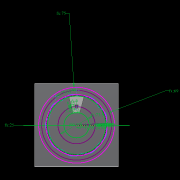
# Autodesk Inventor part: Section_Left_OuterBearing_TBS
Saved by Autodesk Inventor 2022.2 (Build 262287010, 287A)
## iProperties
Created: 2022-05-21
Part Number: Section_Left_OuterBearing_TBS
Material: Generic
Document SubType Name: Modeling
Designer: Árni Þór Þorgeirsson
Density: 1 g/cm^3
Appearance: Default
Author: Árni Þór Þorgeirsson
Autodesk Inventor part; units mm, degrees
ref_plane "YZ Plane" through (0, 0, 0) normal (1, 0, 0) x (0, 1, 0)
ref_plane "XZ Plane" through (0, 0, 0) normal (0, 1, 0) x (-1, 0, 0)
sketch "Sketch1" plane through (0, 0, 0) normal (0, 0, 1) x (1, 0, 0)
  circle A0 centre (0, 0) radius 59.2469 construction
  line L0 (0, 0) -> (59.2469, 0)
  line L1 (0, 0) -> (59.2469, 4.025)
  line L2 (59.2469, 0) -> (59.2469, 4.025)
  circle A1 centre (0, 0) radius 75
  point P0 (56.8, 0)
  dimension "d56" = 59.2469
  dimension "d57" = 4.025
  dimension "d400" = 75
  dimension "d495" = 2.5
  dimension "d496" = 8
  dimension "d531" = 5.5
  dimension "d532" = 5.5
  dimension "d533" = 5.5
  dimension "d537" = 24.5
  dimension "d538" = 3
  dimension "d543" = 5.5
  dimension "d549" = 3
  dimension "d550" = 3
  dimension "d567" = 5.5
  dimension "d568" = 5.5
  constraints: 1 other
sketch "Sketch7" plane through (0, 0, 0) normal (0, 1, 0) x (-1, 0, 0)
  line L0 (0, 0) -> (0, 61.9844)
  line L1 (0, 0) -> (-59.2469, 0) construction
  line L2 (0, 61.9844) -> (-59.2469, 0) construction
  line L3 (0, 61.9844) -> (-64.8494, 0) construction
  line L4 (0, 61.9844) -> (-58.9939, -5.5968) construction
  line L5 (0, 0) -> (0, -61.9844)
  line L6 (0, -61.9844) -> (-59.2469, 0) construction
  line L7 (0, -61.9844) -> (-64.8494, 0) construction
  line L8 (0, -61.9844) -> (-58.9939, 5.5968) construction
  line L9 (-58.9939, 5.5968) -> (-64.8494, 0) construction
  line L10 (-54.1083, 0) -> (-62.8579, -8.363) construction
  line L11 (-54.1083, 0) -> (-38.773, -14.6579) construction
  line L12 (0, -94.3812) -> (0, 132.3969) projected
  line L13 (-75, -5.9919) -> (-75, 6.008)
  line L14 (105, 0) -> (-105, 0) projected
  line L15 (-62.0481, 2.6775) -> (-56.4456, -2.6775) construction
  line L16 (-56.4456, 2.6775) -> (-62.0481, -2.6775) construction
  line L17 (-26.151, -15.9303) -> (-40.3783, -15.9303) construction
  line L18 (-40.3783, -15.9303) -> (-40.3783, -12.7539) construction
  line L19 (-40.3783, -12.7539) -> (-26.151, -12.7539) construction
  line L20 (-26.151, -12.7539) -> (-26.151, -15.9303) construction
  point P0 (-75, 0)
  dimension "Roller_Side_difference" = -0.0002
  dimension "d90" = 61.9844
  dimension "d201" = 75
  dimension "d343" = 92.587
  dimension "d344" = 92.588
  dimension "d367" = 8.1
  constraints: 28 end point, 9 point on line, 3 midpoint, 3 vertical, 2 horizontal, 2 parallel, 2 perpendicular, 1 collinear, 1 symmetric about line, 2 other
  measures "d90" distance of L0.start L0.end
  measures "d201" distance between parallel lines of L5 L13
  measures "d343" angle of L10 L8
  measures "d344" angle of L7 L10
  measures "d367" distance of L3.end L8.end
sketch "Roller1" plane through (0, 0, 0) normal (0, 1, 0) x (-1, 0, 0)
  line L0 (0, 61.9844) -> (-58.9939, -5.5968) construction
  line L1 (0, 61.9844) -> (-64.8494, 0) construction
  line L2 (-54.1083, 0) -> (-38.773, -14.6579) construction
  line L3 (0, -61.9844) -> (-64.8494, 0) construction
  line L4 (-54.0606, 0.0927) -> (-58.9462, -5.5041)
  line L5 (-58.9462, -5.5041) -> (-64.7589, 0.0519)
  line L6 (-64.7589, 0.0519) -> (-59.3884, 5.1851)
  line L7 (-59.3884, 5.1851) -> (-54.0606, 0.0927)
  line L8 (-56.0019, 1.9482) -> (-61.1299, -3.4168)
  line L9 (-61.8526, -2.7261) -> (-56.7246, 2.639)
  point P0 (0, 0)
  dimension "d345" = 0.025
  dimension "d346" = 0.025
  dimension "d347" = 0.1
  dimension "d348" = 0.1
  dimension "d349" = 272.588
  dimension "d350" = 272.587
  dimension "d617" = 0.9997
  constraints: 12 end point, 4 parallel, 3 point on line, 1 midpoint, 1 perpendicular
  measures "d345" distance between parallel lines of L0 L4
  measures "d346" distance between parallel lines of L1 L6
  measures "d347" distance between parallel lines of L3 L5
  measures "d348" distance between parallel lines of L2 L7
  measures "d617" distance between parallel lines of L9 L8
sketch "Roller2" plane through (0, 0, 0) normal (0, 1, 0) x (-1, 0, 0)
  line L0 (0, -61.9844) -> (-58.9939, 5.5968) construction
  line L1 (-54.1083, 0) -> (-62.8579, -8.363) construction
  line L2 (0, -61.9844) -> (-64.8494, 0) construction
  line L3 (0, 61.9844) -> (-64.8494, 0) construction
  line L4 (-58.9956, 5.5606) -> (-54.1429, 0.0016)
  line L5 (-54.1429, 0.0016) -> (-59.4789, -5.0987)
  line L6 (-59.4789, -5.0987) -> (-64.8132, 0)
  line L7 (-64.8132, 0) -> (-58.9956, 5.5606)
  line L8 (-61.9044, 2.7803) -> (-56.8109, -2.5486)
  line L9 (-61.1815, 3.4713) -> (-56.088, -1.8576)
  point P0 (0, 0)
  dimension "d351" = 0.025
  dimension "d352" = 0.025
  dimension "d354" = 0.025
  dimension "d355" = 92.587
  dimension "d356" = 92.588
  dimension "d370" = 0.025
  dimension "d371" = 1
  constraints: 12 end point, 5 parallel, 3 point on line, 1 midpoint, 1 perpendicular
  measures "d351" distance between parallel lines of L0 L4
  measures "d352" distance between parallel lines of L2 L6
  measures "d354" distance between parallel lines of L1 L5
  measures "d355" angle of L5 L4
  measures "d356" angle of L6 L5
  measures "d370" distance from line of L3 L8.start
  measures "d371" distance between parallel lines of L9 L8
sketch "Sketch22" plane through (0, 0, 0) normal (0, 1, 0) x (-1, 0, 0)
  line L0 (-31.756, 8.0215) -> (-17.5287, 8.0215) construction
  line L1 (-17.5287, 8.0215) -> (-17.5287, 4.8451) construction
  line L2 (-17.5287, 4.8451) -> (-31.756, 4.8451) construction
  line L3 (-31.756, 4.8451) -> (-31.756, 8.0215) construction
  point P0 (0, 0)
  dimension "Roller_Side_difference" = -0.0002
  constraints: 2 other
sketch "Sketch2" plane through (0, 0, 0) normal (0, 1, 0) x (-1, 0, 0)
  line L0 (0, 0) -> (0, 59.2469) construction
  line L1 (0, 0) -> (-59.2469, 0) projected
  line L2 (0, 0) -> (0, -59.2469)
  line L3 (0, -59.2469) -> (-59.2469, 0) construction
  line L4 (0, 59.2469) -> (-59.2469, 0) construction
  line L5 (-50.4879, 53.555) -> (0, 59.2469) construction
  line L6 (-29.7354, 7.189) -> (0, 59.2469) construction
  line L7 (-29.7354, 7.189) -> (0, -59.2469) construction
  line L8 (-48.8381, -26.254) -> (0, -59.2469) construction
  point P0 (-40.4258, 18.8211)
  constraints: 16 end point, 3 point on line, 1 perpendicular, 1 symmetric about line, 1 vertical
sketch "Sketch23" plane through (0, 0, 0) normal (0, 1, 0) x (-1, 0, 0)
  line L0 (0, -61.9844) -> (-58.9939, 5.5968) construction
  line L1 (0, -61.9844) -> (-64.8494, 0) construction
  line L2 (0, 61.9844) -> (-58.9939, -5.5968) construction
  line L3 (-58.9939, 5.5968) -> (-64.8494, 0) construction
  line L4 (0, 61.9844) -> (-64.8494, 0) construction
  line L5 (-58.9939, 5.5968) -> (-58.9939, -5.5968) construction
  line L6 (105, 0) -> (-105, 0) projected
  line L7 (-57.6514, 4.0968) -> (-54.1326, 0.0658)
  line L8 (-54.1326, -0.0658) -> (-57.6514, -4.0968)
  line L9 (-60.5995, 4.0968) -> (-64.81, 0.0723)
  line L10 (-64.81, -0.0723) -> (-60.5995, -4.0968)
  arc A0 (-64.81, 0.0723) -> (-64.81, -0.0723) centre (-64.7409, 0) ccw
  arc A1 (-54.1326, -0.0658) -> (-54.1326, 0.0658) centre (-54.2079, 0) ccw
  line L11 (-57.6514, 4.0968) -> (-57.6514, 5.5968)
  line L12 (-57.6514, 5.5968) -> (-25, 5.5968)
  line L13 (-25, 5.5968) -> (-25, -5.5968)
  line L14 (-25, -5.5968) -> (-57.6514, -5.5968)
  line L15 (-57.6514, -5.5968) -> (-57.6514, -4.0968)
  line L16 (-60.5995, 4.0968) -> (-60.5995, 5.5968)
  line L17 (-60.5995, 5.5968) -> (-75, 5.5968)
  line L18 (-75, 5.5968) -> (-75, -5.5968)
  line L19 (-60.5995, -4.0968) -> (-60.5995, -5.5968)
  line L20 (-60.5995, -5.5968) -> (-75, -5.5968)
  line L21 (-58.9939, 5.5968) -> (-58.9939, 5.5968)
  line L22 (-58.9939, -5.5968) -> (-58.9939, -5.5968)
  line L23 (0, -94.3812) -> (0, 132.3969) projected
  line L24 (-64.8856, 0) -> (-75, 0)
  point P0 (0, 0)
  point P1 (-54.0752, 0)
  point P2 (-64.8409, 0)
  point P3 (-75, 0)
  dimension "d378" = 90
  dimension "d379" = 0.1
  dimension "d380" = 0.025
  dimension "d381" = 0.025
  dimension "d382" = 0.025
  dimension "d383" = 0.025
  dimension "d384" = 11.1935
  dimension "d385" = 0
  dimension "d386" = 0
  dimension "d391" = 25
  dimension "d392" = 75
  dimension "d393" = 1.5
  dimension "d394" = 1.5
  dimension "d395" = 1.5
  dimension "d396" = 1.5
  constraints: 36 end point, 10 point on line, 9 vertical, 4 horizontal, 4 parallel, 4 point on circle, 4 tangent, 2 centre point, 1 equal radius, 1 midpoint
  measures "d378" angle of L6 L5
  measures "d379" radius of A0
  measures "d380" distance between parallel lines of L9 L4
  measures "d381" distance between parallel lines of L10 L1
  measures "d382" distance between parallel lines of L0 L7
  measures "d383" distance between parallel lines of L2 L8
  measures "d384" distance of L0.end L2.end
  measures "d385" distance of L2.end L22.end
  measures "d386" distance of L0.end L21.end
  measures "d391" distance between parallel lines of L23 L13
  measures "d392" distance between parallel lines of L18 L23
  measures "d393" distance of L9.start L16.end
  measures "d394" distance of L7.start L11.end
  measures "d395" distance of L14.end L8.end
  measures "d396" distance of L10.end L19.end
revolve "RevRoller1" [suppressed]
fillet "Fillet1" [suppressed]
sketch "Sketch48" plane through (56.7246, 0, 2.639) normal (-0.691, 0, 0.7229) x (0.7229, 0, 0.691)
  line L0 (-2.5, 0.25) -> (2.5, 0.25)
  line L1 (2.5, 0.25) -> (2.5, -0.25)
  line L2 (2.5, -0.25) -> (-2.5, -0.25)
  line L3 (-2.5, -0.25) -> (-2.5, 0.25)
  line L4 (-2.5, 0.25) -> (2.5, -0.25) construction
  line L5 (2.5, 0.25) -> (-2.5, -0.25) construction
  line L6 (-0.25, -2.5) -> (0.25, -2.5)
  line L7 (0.25, -2.5) -> (0.25, 2.5)
  line L8 (0.25, 2.5) -> (-0.25, 2.5)
  line L9 (-0.25, 2.5) -> (-0.25, -2.5)
  line L10 (-0.25, -2.5) -> (0.25, 2.5) construction
  line L11 (0.25, -2.5) -> (-0.25, 2.5) construction
  point P0 (-42.8293, 0)
  point P1 (0, 0)
  point P2 (-0.25, 0.25)
  point P3 (-0.25, -0.25)
  point P4 (0.25, -0.25)
  point P5 (0.25, 0.25)
  dimension "d621" = 5
  dimension "d622" = 0.5
  dimension "d623" = 0.5
  dimension "d624" = 5
  constraints: 24 end point, 4 midpoint, 4 parallel, 2 horizontal, 2 perpendicular
  measures "d621" distance of L1.end L2.end
  measures "d622" distance of L0.end L1.end
  measures "d623" distance of L8.end L7.end
  measures "d624" distance of L7.end L6.end
extrude "Extrusion39" [suppressed]
sketch "Sketch40" plane through (0, 0, -5.231) normal (0, 0, -1) x (-1, 0, 0)
  circle A0 centre (53.5, 0) radius 2.75 projected
  circle A1 centre (0, 0) radius 53.5 projected
  point P0 (53.4293, 2.7491)
  point P1 (53.4293, -2.7491)
  dimension "d585" = 8
  dimension "d587" = 1.75
  dimension "d589" = 3
  dimension "d592" = 2
  dimension "d593" = 12
  dimension "d594" = 12
  dimension "d611" = 360
  constraints: 18 point on circle, 10 centre point, 8 end point, 2 midpoint, 1 horizontal alignment, 1 vertical, 29 other
  measures "d589" diameter of A1
pattern_circular "Circular Pattern13" [suppressed]
feature "Move Body7" [suppressed]
revolve "Revolution13" [suppressed]
fillet "Fillet3" [suppressed]
pattern_circular "Circular Pattern14" [suppressed]
feature "Move Body6" [suppressed]
revolve "Revolution14" add sketch "Sketch23" angle 360 about axis through (0, 0, -10) along (0, 0, 1) contours A1 L7 L11 L12 L13 L6 | L6 L13 L14 L15 L8 A1
revolve "OuterRim_Top2" [suppressed]
revolve "OuterRim_Bottom2" [suppressed]
ref_plane "Work Plane8" through (0, 0, 20) normal (0, 0, 1) x (1, 0, 0)
sketch "Sketch49" plane through (0, 0, 20) normal (0, 0, 1) x (1, 0, 0)
  circle A0 centre (0, 0) radius 75 projected
  circle A1 centre (0, 0) radius 60.5995 projected
  circle A2 centre (0, 0) radius 57.6514 projected
  circle A3 centre (0, 0) radius 25 projected
  circle A4 centre (0, 0) radius 69
  circle A5 centre (0, 0) radius 36.75
  point P0 (0, 69)
  point P1 (0, 36.75)
  point P2 (-40.5572, 55.8222)
  dimension "d629" = 69
  dimension "d630" = 73.5
  dimension "d649" = 36
  constraints: 2 coincident, 2 vertical alignment, 6 other
sketch "Sketch50" plane through (0, 0, 5.5968) normal (0, 0, 1) x (1, 0, 0)
  point P0 (0, 0)
  point P1 (0, 69)
sketch "Sketch51" plane through (0, 0, -5.5968) normal (0, 0, -1) x (-1, 0, 0)
  circle A0 centre (0, 0) radius 75 projected
  circle A1 centre (0, 69) radius 2.75
  circle A2 centre (0, 69) radius 1.5
  circle A3 centre (-40.5572, 55.8222) radius 3.5
  circle A4 centre (-40.5572, 55.8222) radius 2
  dimension "d633" = 36
  dimension "d635" = 5.5
  dimension "d636" = 3
  dimension "d637" = 7
  dimension "d638" = 4
  constraints: 4 centre point, 4 coincident, 2 other
  measures "d635" diameter of A1
  measures "d636" diameter of A2
  measures "d637" diameter of A3
  measures "d638" diameter of A4
extrude "Extrusion40" [suppressed]
extrude "Extrusion41" [suppressed]
extrude "Extrusion42" [suppressed]
extrude "Extrusion43" [suppressed]
sketch "Sketch52" plane through (0, 0, 5.5968) normal (0, 0, 1) x (1, 0, 0)
  circle A0 centre (0, 69) radius 1.5
  circle A1 centre (-40.5572, 55.8222) radius 2
  line L0 (2.75, 67.4123) -> (0, 65.8246)
  line L1 (0, 65.8246) -> (-2.75, 67.4123)
  line L2 (-2.75, 67.4123) -> (-2.75, 70.5877)
  line L3 (-2.75, 70.5877) -> (0, 72.1754)
  line L4 (0, 72.1754) -> (2.75, 70.5877)
  line L5 (2.75, 70.5877) -> (2.75, 67.4123)
  circle A2 centre (0, 0) radius 75 projected
  line L6 (-39.2656, 58.7231) -> (-37.3992, 56.1541)
  line L7 (-36.5379, 56.2446) -> (-38.1817, 52.5526)
  line L8 (-38.1817, 52.5526) -> (-42.201, 52.1301)
  line L9 (-42.201, 52.1301) -> (-44.5765, 55.3997)
  line L10 (-44.5765, 55.3997) -> (-42.9327, 59.0918)
  line L11 (-42.9327, 59.0918) -> (-38.9134, 59.5142)
  line L12 (-38.9134, 59.5142) -> (-36.5379, 56.2446)
  dimension "d651" = 3
  dimension "d652" = 4
  dimension "d655" = 36
  dimension "d657" = 7
  dimension "d658" = 5.5
  constraints: 26 end point, 4 coincident, 2 centre point, 1 parallel, 30 other
  measures "d651" diameter of A0
  measures "d652" diameter of A1
  measures "d657" distance between parallel lines of L12 L9
  measures "d658" distance between parallel lines of L5 L2
extrude "Extrusion44" [suppressed]
extrude "Extrusion45" [suppressed]
extrude "Extrusion46" [suppressed]
extrude "Extrusion47" [suppressed]
pattern_circular "Circular Pattern32" [suppressed]
pattern_circular "Circular Pattern33" [suppressed]
sketch "Sketch57" plane through (0, 0, -5.5968) normal (0, 0, -1) x (-1, 0, 0)
  line L0 (-3.175, 39.925) -> (3.175, 39.925)
  line L1 (3.175, 39.925) -> (3.175, 33.575)
  line L2 (3.175, 33.575) -> (-3.175, 33.575)
  line L3 (-3.175, 33.575) -> (-3.175, 39.925)
  line L4 (-3.175, 39.925) -> (3.175, 33.575) construction
  line L5 (3.175, 39.925) -> (-3.175, 33.575) construction
  ellipse E0 centre (0, 36.75) end of major axis (6.4, 36.75) minor radius 5.45
  point P0 (0, 0)
  dimension "d694" = 6.35
  dimension "d695" = 6.35
  dimension "d696" = 6.4
  dimension "d697" = 5.45
  constraints: 12 end point, 2 midpoint, 2 parallel, 1 centre point, 1 coincident, 1 horizontal, 1 perpendicular, 1 other
  measures "d694" distance of L1.end L2.end
  measures "d695" distance of L0.end L1.end
extrude "Extrusion50" cut sketch "Sketch57" against normal blind 11.194 contours L0 L1 L2 L3
extrude "Extrusion51" cut sketch "Sketch57" against normal blind 8.194 contours L0 L1 L2 L3 | E0
pattern_circular "Circular Pattern34" count 6 over 360 about axis through (0, 0, -4.8468) along (0, 0, 1) of "Extrusion50", "Extrusion51"
ref_plane "Work Plane9" through (0, 0, -25) normal (0, 0, 1) x (1, 0, 0)
sketch "Sketch58" plane through (0, 0, -25) normal (0, 0, 1) x (1, 0, 0)
  line L0 (0, 0) -> (0, 94.5267)
  line L1 (0, 94.5267) -> (0, 0)
  line L2 (0, 0) -> (-27.705, 103.3964)
  line L3 (0, 0) -> (25.7729, 96.1857)
  circle A0 centre (0, 0) radius 95.9893
  point P0 (-24.8439, 92.7185)
  point P1 (24.8439, 92.7185)
  dimension "d706" = 15
  dimension "d707" = 15
  constraints: 8 end point, 1 centre point, 1 coincident, 1 collinear, 1 vertical
  measures "d706" angle of L2 L0
  measures "d707" angle of L0 L3
extrude "Extrusion52" cut sketch "Sketch58" along normal through all contours L3 A0 L2 picked at (37.9953, -51.2872)
equation "\"Roller_Side_difference\" = -0.000942deg"
equation "\"Cycloid_Top_Plate_Fasner_Inner\" = 61.25"
equation "\"Cycloid_Top_Plate_Fasner_Outer\" = 85.75"
equation "\"Roller_Hole_Radius\" = 1"
equation "\"Distance_To_Bearing\" = 85.74529"
equation "\"d514\" = 0.2"
equation "\"Machine_Screw_4mm_Head_Dept\" = 4"
equation "\"Machine_Screw_4mm_Head_Diameter\" = 7"
equation "\"Machine_Screw_4mm_HexNut_Thickness\" = 3"
equation "\"Machine_Screw_4mm_HexNut_Width\" = 6.9"
equation "\"Machine_Screw_4mm_Length\" = 8"
equation "\"Fastner_4mm_Hex_Nut_Width\" = 7"
equation "\"Fastner_4mm_Screw_Diameter\" = 4"
equation "\"Fastner_4mm_Screw_Head_Diameter\" = 7"
equation "\"Fastner_4mm_Hex_Nut_Hole_Dept\" = 3.19352"
equation "\"Fastner_4mm_Screw_Head_Hole_Dept\" = 4"
body "Solid1"
body "Solid5"
